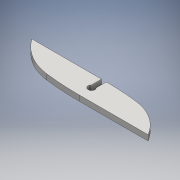
# Autodesk Inventor part: balancin
Saved by Autodesk Inventor 2016 (Build 200138000, 138)
## iProperties
Created: 2016-09-20
Part Number: balancin
Material: Madera (abedul)
Document SubType Name: Modeling
Designer: i95sa
Density: 0.55 g/cm^3
Appearance: Suave - Blanco
Author: i95sa
Autodesk Inventor part; units mm, degrees
ref_plane "YZ Plane" through (0, 0, 0) normal (1, 0, 0) x (0, 1, 0)
ref_plane "XZ Plane" through (0, 0, 0) normal (0, 1, 0) x (-1, 0, 0)
ref_plane "XY Plane" through (0, 0, 0) normal (0, 0, 1) x (1, 0, 0)
sketch "Boceto1" plane through (0, 0, 0) normal (0, 0, 1) x (1, 0, 0)
  arc A0 (-2.2913, 1) -> (2.2913, 1) centre (0, 0) ccw
  arc A1 (-25.0314, -7.4961) -> (0, -9) centre (-0.6579, 189.118) ccw
  arc A2 (24.9974, 7.5103) -> (2.2913, 8.9972) centre (0.9036, -186.3114) ccw
  line L0 (0, -9) -> (50, -9)
  line L1 (-2.2913, 9) -> (-52.2913, 9)
  arc A3 (-52.2913, 9) -> (-25.0314, -7.4961) centre (-20.234, 31.2032) ccw
  arc A4 (50, -9) -> (24.9974, 7.5103) centre (20.8341, -25.9812) ccw
  line L2 (-1.75, 9) -> (-1.75, 1)
  line L3 (1.75, 8.9972) -> (1.75, 1)
  line L4 (1.75, 1) -> (2.2913, 1)
  line L5 (-1.75, 1) -> (-2.2913, 1)
  line L6 (-1.75, 9) -> (-2.2913, 9)
  line L7 (1.75, 8.9972) -> (2.2913, 8.9972)
  dimension "d0" = 5
  dimension "d31" = 50
  dimension "d32" = 50
  constraints: 16 end point, 11 point on circle, 5 centre point, 2 collinear, 2 tangent, 1 coincident, 1 horizontal, 1 parallel, 1 perpendicular, 1 point on line
  measures "d0" diameter of A0
  measures "d31" distance of L0.start L0.end
  measures "d32" distance of L1.start L1.end
extrude "Extrusión3" add sketch "Boceto1" along normal blind 4
